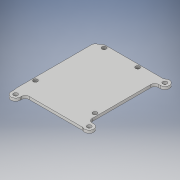
# Autodesk Inventor part: ArduinoPlate
Saved by Autodesk Inventor 2018 (Build 220112000, 112)
## iProperties
Created: 2019-10-01
Part Number: ArduinoPlate
Material: Generic
Document SubType Name: Modeling
Designer: anirudh
Density: 1 g/cm^3
Appearance: Default
Author: anirudh
Autodesk Inventor part; units mm, degrees
ref_plane "YZ Plane" through (0, 0, 0) normal (1, 0, 0) x (0, 1, 0)
ref_plane "XZ Plane" through (0, 0, 0) normal (0, 1, 0) x (-1, 0, 0)
ref_plane "XY Plane" through (0, 0, 0) normal (0, 0, 1) x (1, 0, 0)
sketch "Sketch1" plane through (0, 0, 0) normal (0, 1, 0) x (-1, 0, 0)
  line L0 (53.34, 2.2324) -> (53.34, -63.8076)
  line L1 (53.34, -63.8076) -> (50.8, -63.8076)
  line L2 (48.26, -66.3476) -> (15.494, -66.3476)
  line L3 (50.8, -63.8076) -> (48.26, -66.3476)
  line L4 (0, -60.2503) -> (0, -4.8703)
  circle A0 centre (17.78, -63.8076) radius 1.75
  circle A1 centre (45.72, -63.8076) radius 1.75
  circle A2 centre (2.54, -13.0076) radius 1.75
  circle A3 centre (50.8, -11.7376) radius 1.75
  circle A4 centre (-4.5731, -1.0603) radius 1.75
  circle A5 centre (-4.5731, -1.0603) radius 1.75
  circle A6 centre (49.1069, 6.4197) radius 1.75
  circle A7 centre (49.1069, 6.4197) radius 1.75
  circle A8 centre (-4.5731, -64.0603) radius 1.75
  circle A9 centre (-4.5731, -64.0603) radius 1.75
  arc A10 (-4.5731, -60.2503) -> (-1.5261, -66.3476) centre (-4.5731, -64.0603) ccw
  arc A11 (-2.6564, 2.2324) -> (-4.5731, -4.8703) centre (-4.5731, -1.0603) ccw
  arc A12 (52.9169, 6.4197) -> (45.2969, 6.4197) centre (49.1069, 6.4197) ccw
  line L5 (0, 2.2324) -> (-2.6564, 2.2324)
  line L6 (-4.5731, -4.8703) -> (0, -4.8703)
  line L7 (15.494, -66.3476) -> (-1.5261, -66.3476)
  line L8 (-4.5731, -60.2503) -> (0, -60.2503)
  line L9 (45.2969, 6.4197) -> (45.2969, 2.2324)
  line L10 (52.9169, 6.4197) -> (52.9169, 2.2324)
  line L11 (0, 2.2324) -> (45.2969, 2.2324)
  line L12 (52.9169, 2.2324) -> (53.34, 2.2324)
  dimension "d2" = 3.5
  dimension "d3" = 3.5
  dimension "d9" = 7.62
  dimension "d10" = 7.62
  constraints: 26 end point, 13 centre point, 6 coincident, 6 perpendicular, 6 point on circle, 4 tangent, 1 horizontal, 1 parallel, 1 vertical
  measures "d2" diameter of A2
  measures "d3" diameter of A3
  measures "d9" diameter of A10
  measures "d10" diameter of A11
extrude "Extrusion1" add sketch "Sketch1" along normal blind 2.286
fillet "Fillet1" radius 3.175 6 edges at (-52.9169, 1.143, 2.2324) (-45.2969, 1.143, 2.2324) (2.6564, 1.143, 2.2324) (0, 1.143, -4.8703) (0, 1.143, -60.2503) (1.5261, 1.143, -66.3476)
fillet "Fillet2" radius 3.175 3 edges at (-48.26, 1.143, -66.3476) (-50.8, 1.143, -63.8076) (-53.34, 1.143, -63.8076)
body "Solid1"
